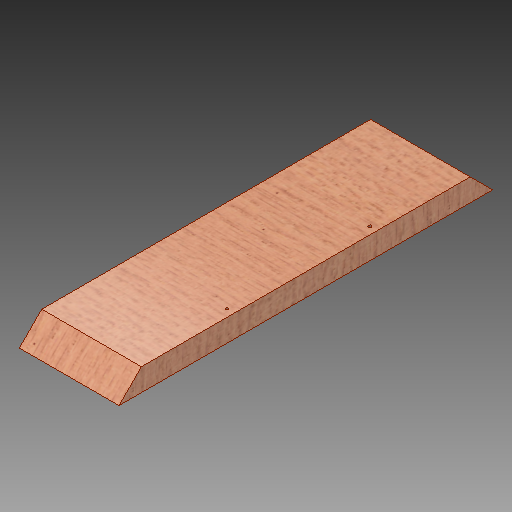
# Autodesk Inventor part: Front
Saved by Autodesk Inventor 2019.3 (Build 233278000, 278)
## iProperties
Created: 2019-01-12
Part Number: Front
Material: Holz (Eiche)
Document SubType Name: Modeling
Designer: Jonas
Density: 0.76 g/cm^3
Appearance: Weißeiche - natur - mittlerer Glanz
Author: Jonas
Autodesk Inventor part; units mm, degrees
ref_plane "YZ Plane" through (0, 0, 0) normal (1, 0, 0) x (0, 1, 0)
ref_plane "XZ Plane" through (0, 0, 0) normal (0, 1, 0) x (-1, 0, 0)
ref_plane "XY Plane" through (0, 0, 0) normal (0, 0, 1) x (1, 0, 0)
sketch "Skizze1" plane through (0, 0, 0) normal (0, 1, 0) x (-1, 0, 0)
  line L0 (35.9259, 133.0751) -> (-44.0741, 133.0751)
  line L1 (-44.0741, 133.0751) -> (-44.0741, -166.9249)
  line L2 (-44.0741, -166.9249) -> (35.9259, -166.9249)
  line L3 (35.9259, -166.9249) -> (35.9259, 133.0751)
  point P0 (0, 0)
  dimension "d0" = 80
  dimension "d1" = 300
  constraints: 8 end point, 2 parallel, 1 horizontal, 1 perpendicular
  measures "d0" distance of L0.start L0.end
  measures "d1" distance of L2.end L0.start
extrude "Extrusion1" add sketch "Skizze1" along normal blind 18
chamfer "Fase1" distance 18 angle 45 1 edges at (4.0741, 18, 133.0751)
chamfer "Fase2" distance 18 angle 45 1 edges at (4.0741, 18, -166.9249)
sketch "Skizze2" plane through (0, 18, 0) normal (0, 1, 0) x (1, 0, 0)
  point P0 (38.0741, -40.5751)
hole "Bohrung1" at (38.0741, 18, 40.5751) direction (0, -1, 0) diameter 2.013 depth 8 tip angle 120 thread size "M2.5x0.45" class "6H" standard "ISO Metric profile"
sketch "Skizze3" plane through (0, 18, 0) normal (0, 1, 0) x (1, 0, 0)
  point P0 (38.0741, 74.4249)
hole "Bohrung3" at (38.0741, 18, -74.4249) direction (0, -1, 0) diameter 2.459 depth 8 tip angle 120 thread size "M3x0.5" class "6H" standard "ISO Metric profile"
